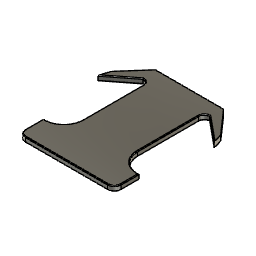
lfr2 design (Autodesk Fusion 360 design; units mm, degrees)
Autodesk Fusion 360 part; units mm, degrees
sketch "Sketch1" plane through (0, 0, 0) normal (0, 0, 1) x (1, 0, 0)
  line L0 (-50.0247, -1.0934) -> (49.9753, -1.0934)
  line L1 (-50.0192, -21.0934) -> (-47.9925, -21.0934)
  line L2 (-39.9925, -29.0934) -> (-39.9925, -117.0004)
  line L3 (-67.9925, -145.0004) -> (-69.9997, -145.0004)
  line L4 (-69.9997, -145.0004) -> (-69.9997, -171.0934)
  line L5 (48, -19.4614) -> (48.0075, -19.4614)
  line L6 (40.0075, -27.4614) -> (40.0075, -116.9996)
  line L7 (68.0075, -144.9996) -> (69.9997, -144.9996)
  line L8 (69.9997, -144.9996) -> (69.9997, -171.0934)
  line L9 (59.9997, -181.0934) -> (-59.9997, -181.0934)
  arc A0 (-67.9925, -145.0004) -> (-39.9925, -117.0004) centre (-67.9925, -117.0004) ccw
  arc A1 (40.0075, -116.9996) -> (68.0075, -144.9996) centre (68.0075, -116.9996) ccw
  arc A2 (59.9997, -181.0934) -> (69.9997, -171.0934) centre (59.9997, -171.0934) ccw
  arc A3 (-69.9997, -171.0934) -> (-59.9997, -181.0934) centre (-59.9997, -171.0934) ccw
  arc A4 (48.0075, -19.4614) -> (40.0075, -27.4614) centre (48.0075, -27.4614) ccw
  arc A5 (-39.9925, -29.0934) -> (-47.9925, -21.0934) centre (-47.9925, -29.0934) ccw
  line L10 (-50.0247, -1.0934) -> (-79.9919, -34.9935)
  line L11 (49.9753, -1.0934) -> (80.1359, -35.4644)
  line L12 (-79.9919, -34.9935) -> (-84.9925, -50.0042)
  line L13 (-84.9925, -50.0042) -> (-47.9925, -21.0934)
  line L14 (80.1359, -35.4644) -> (85, -50)
  line L15 (85, -50) -> (48, -19.4614)
  dimension "d4" = 100
  dimension "d5" = 20
  dimension "d6" = 80
  dimension "d8" = 28
  dimension "d9" = 28
  dimension "d11" = 10
  dimension "d12" = 10
  dimension "d13" = 8
  dimension "d14" = 8
  dimension "d19" = 180
  dimension "d31" = 37
  dimension "d32" = 37
  constraint horizontal L0
  constraint perpendicular L1 L2
  constraint perpendicular L2 L3
  constraint perpendicular L3 L4
  constraint perpendicular L5 L6
  constraint perpendicular L6 L7
  constraint perpendicular L7 L8
  constraint perpendicular L4 L9
  constraint tangent L3 A0
  constraint tangent L2 A0
  constraint tangent L6 A1
  constraint tangent L7 A1
  constraint tangent L4 A3
  constraint tangent L9 A3
  constraint tangent L9 A2
  constraint tangent L8 A2
  constraint tangent L1 A5
  constraint tangent L2 A5
  constraint tangent L5 A4
  constraint tangent L6 A4
  measures "d4" distance of L0.start L0.end
  measures "d5" distance of L0.start L1.start
  measures "d6" distance of L2 L6
  measures "d8" radius of A0
  measures "d9" radius of A1
  measures "d11" radius of A3
  measures "d12" radius of A2
  measures "d13" radius of A5
  measures "d14" radius of A4
  measures "d19" distance of L0 L9
  measures "d31" horizontal distance of L1.end L12.end
  measures "d32" horizontal distance of L5.start L14.end
extrude "Extrude2" add sketch "Sketch1" along normal mid plane 7.5
fillet "Fillet5" radius 1 26 edges at (-69.9997, -158.0469, 3.75) (-67.0708, -178.1645, 3.75) (0, -181.0934, 3.75) (67.0708, -178.1645, 3.75) (69.9997, -158.0465, 3.75) (69.9997, -158.0465, -3.75) (67.0708, -178.1645, -3.75) (0, -181.0934, -3.75) (-67.0708, -178.1645, -3.75) (-69.9997, -158.0469, -3.75) (-42.3357, -23.4365, 3.75) (-39.9925, -73.0469, 3.75) (-48.1935, -136.7994, 3.75) (-68.9961, -145.0004, 3.75) (69.0036, -144.9996, 3.75) (48.2085, -136.7986, 3.75) (40.0075, -72.2305, 3.75) (42.348, -21.8072, 3.75) (42.348, -21.8072, -3.75) (40.0075, -72.2305, -3.75) (48.2085, -136.7986, -3.75) (69.0036, -144.9996, -3.75) (-68.9961, -145.0004, -3.75) (-48.1935, -136.7994, -3.75) (-39.9925, -73.0469, -3.75) (-42.3357, -23.4365, -3.75)
fillet "Fillet6" radius 1 4 edges at (-65.9024, -35.0877, 3.75) (-65.9024, -35.0877, -3.75) (65.9375, -34.2664, -3.75) (65.9375, -34.2664, 3.75)
